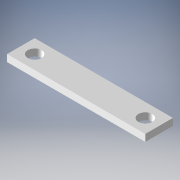
# Autodesk Inventor part: 15102898-16-P-0224
Saved by Autodesk Inventor 2017 (Build 210142000, 142)
## iProperties
Created: 2016-11-06
Part Number: 15102898-16-P-0224
Material: Generic
Document SubType Name: Modeling
Designer: gus
Density: 1 g/cm^3
Appearance: Default
Author: gus
Autodesk Inventor part; units mm, degrees
ref_plane "YZ Plane" through (0, 0, 0) normal (1, 0, 0) x (0, 1, 0)
ref_plane "XZ Plane" through (0, 0, 0) normal (0, 1, 0) x (-1, 0, 0)
ref_plane "XY Plane" through (0, 0, 0) normal (0, 0, 1) x (1, 0, 0)
sketch "Sketch1" plane through (0, 0, 0) normal (0, 1, 0) x (-1, 0, 0)
  line L0 (0, 0) -> (57.15, 0)
  line L1 (57.15, 0) -> (57.15, -19.05)
  line L2 (57.15, -19.05) -> (0, -19.05)
  line L3 (0, -19.05) -> (0, 0)
  circle A0 centre (6.35, -9.525) radius 3.175
  circle A1 centre (50.8, -9.525) radius 3.175
  circle A2 centre (31.75, -9.525) radius 4.7625
  dimension "d0" = 57.15
  dimension "d1" = 19.05
  dimension "d2" = 6.35
  dimension "d3" = 6.35
  dimension "d4" = 9.525
  dimension "d5" = 6.35
  dimension "d6" = 6.35
  dimension "d7" = 9.525
  dimension "d12" = 9.525
  dimension "d13" = 31.75
  dimension "d14" = 9.525
  constraints: 8 end point, 3 centre point, 2 parallel, 1 horizontal, 1 perpendicular
  measures "d0" distance of L1.end L2.end
  measures "d1" distance of L2.end L0.start
  measures "d2" diameter of A0
  measures "d3" diameter of A1
  measures "d4" distance from line of L2 A1.centre
  measures "d5" distance from line of L1 A1.centre
  measures "d6" distance from line of L3 A0.centre
  measures "d7" distance from line of L2 A0.centre
  measures "d12" diameter of A2
  measures "d13" distance from line of L3 A2.centre
  measures "d14" distance from line of L0 A2.centre
extrude "Extrusion1" add sketch "Sketch1" along normal blind 3.175 contours L0 L1 L2 L3 | A2
extrude "Extrusion2" cut sketch "Sketch1" along normal blind 3.175 contours A2
body "Solid1"
